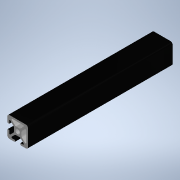
# Autodesk Inventor part: ITEM_20x20_N2_180mm
Saved by Autodesk Inventor 2022 (Build 260153000, 153)
## iProperties
Part Number: ITEM_20x20_N2_180mm
Material: Generic
Document SubType Name: Modeling
Designer: Alexander Fritzsche
Appearance: Default
Author: Alexander Fritzsche
Autodesk Inventor part; units mm, degrees
ref_plane "YZ Plane" through (0, 0, 0) normal (1, 0, 0) x (0, 1, 0)
ref_plane "XZ Plane" through (0, 0, 0) normal (0, 1, 0) x (-1, 0, 0)
ref_plane "XY Plane" through (0, 0, 0) normal (0, 0, 1) x (1, 0, 0)
sketch "Sketch1" plane through (0, 0, 0) normal (0, 0, 1) x (1, 0, 0)
  circle A0 centre (0, 0) radius 2.15
  line L0 (-6.9272, 8.2) -> (-2.3772, 3.65)
  line L1 (-2.3772, 3.65) -> (2.3772, 3.65)
  line L2 (2.3772, 3.65) -> (6.9272, 8.2)
  line L3 (8.2, 6.9272) -> (3.65, 2.3772)
  line L4 (3.65, 2.3772) -> (3.65, -2.3772)
  line L5 (3.65, -2.3772) -> (8.2, -6.9272)
  line L6 (10, -10) -> (2.5, -10)
  line L7 (2.5, -10) -> (2.5, -8.2)
  line L8 (2.5, -8.2) -> (6.9272, -8.2)
  line L9 (6.9272, -8.2) -> (2.3772, -3.65)
  line L10 (2.3772, -3.65) -> (-2.3772, -3.65)
  line L11 (-2.3772, -3.65) -> (-6.9272, -8.2)
  line L12 (-6.9272, -8.2) -> (-2.5, -8.2)
  line L13 (-2.5, -8.2) -> (-2.5, -10)
  line L14 (-2.5, -10) -> (-10, -10)
  line L15 (-10, -10) -> (-10, -2.5)
  line L16 (-10, -2.5) -> (-8.2, -2.5)
  line L17 (-8.2, -2.5) -> (-8.2, -6.9272)
  line L18 (-8.2, -6.9272) -> (-3.65, -2.3772)
  line L19 (-3.65, -2.3772) -> (-3.65, 2.3772)
  line L20 (-3.65, 2.3772) -> (-8.2, 6.9272)
  line L21 (-8.2, 6.9272) -> (-8.2, 2.5)
  line L22 (-8.2, 2.5) -> (-10, 2.5)
  line L23 (-10, 2.5) -> (-10, 10)
  line L24 (0, 0) -> (-30.8654, 30.8654)
  line L25 (0, 0) -> (30.8654, 30.8654)
  line L26 (0, 0) -> (42.5392, 0)
  line L27 (0, 0) -> (0, 44.3419)
  line L28 (-10, 10) -> (10, 10)
  line L29 (-6.9272, 8.2) -> (6.9272, 8.2)
  line L30 (8.2, 6.9272) -> (8.2, -6.9272)
  line L31 (10, -10) -> (10, 10)
  dimension "d0" = 45
  dimension "d1" = 90
  dimension "Durchmesser_Loch" = 4.3
  dimension "Wandstaerke" = 1.8
  dimension "d3" = 1.8
  dimension "Breite_Schiene" = 5
  dimension "d16" = 1.8
  dimension "Tiefe_Schiene" = 6.35
  dimension "Breite" = 20
  dimension "d19" = 1.8
  dimension "d20" = 5
  constraints: 64 end point, 10 parallel, 9 point on line, 8 perpendicular, 4 collinear, 3 vertical, 2 horizontal, 1 centre point, 1 coincident, 8 other
  measures "d0" angle of L25 L26
  measures "d1" angle of L25 L24
  measures "Durchmesser_Loch" diameter of A0
  measures "Wandstaerke" distance between parallel lines of L0 L20
  measures "d3" distance between parallel lines of L11 L18
  measures "Breite_Schiene" distance between parallel lines of L16 L22
  measures "d16" distance between parallel lines of L28 L29
  measures "Tiefe_Schiene" distance between parallel lines of L28 L1
  measures "Breite" distance between parallel lines of L6 L28
  measures "d19" distance of L21.end L22.end
  measures "d20" distance between parallel lines of L7 L13
extrude "Extrusion1" add sketch "Sketch1" along normal mid plane 140 contours L26 L4 L5 L30 L31 L6 L7 L8 L9 L10 L11 L12 L13 L14 L15 L16 L17 L18 L19 L20 L21 L22 L23 L24 A0 | A0 L25 L31 L26 L30 L3 L4 | A0 L27 L1 L2 L29 L28 L25 | L24 L28 L27 L29 L0 L1 A0
fillet "Fillet1" radius 2 4 edges at (10, 10, 0) (-10, 10, 0) (10, -10, 0) (-10, -10, 0)
fillet "Fillet2" radius 0.2 4 edges at (-2.5, -8.2, 0) (-8.2, -2.5, 0) (-8.2, 2.5, 0) (2.5, -8.2, 0)
fillet "Fillet3" radius 0.7 12 edges at (2.5, -10, 0) (-2.5, -10, 0) (-10, -2.5, 0) (-10, 2.5, 0) (-6.9272, -8.2, 0) (-8.2, -6.9272, 0) (6.9272, -8.2, 0) (-8.2, 6.9272, 0) (-6.9272, 8.2, 0) (6.9272, 8.2, 0) (8.2, 6.9272, 0) (8.2, -6.9272, 0)
fillet "Fillet4" radius 2 8 edges at (-3.65, 2.3772, 0) (2.3772, -3.65, 0) (-2.3772, -3.65, 0) (-3.65, -2.3772, 0) (-2.3772, 3.65, 0) (2.3772, 3.65, 0) (3.65, 2.3772, 0) (3.65, -2.3772, 0)
equation "\"d3\" = Wandstaerke"
equation "\"d16\" = Wandstaerke"
equation "\"d19\" = Wandstaerke"
equation "\"d20\" = Breite_Schiene"
body "Solid1"
